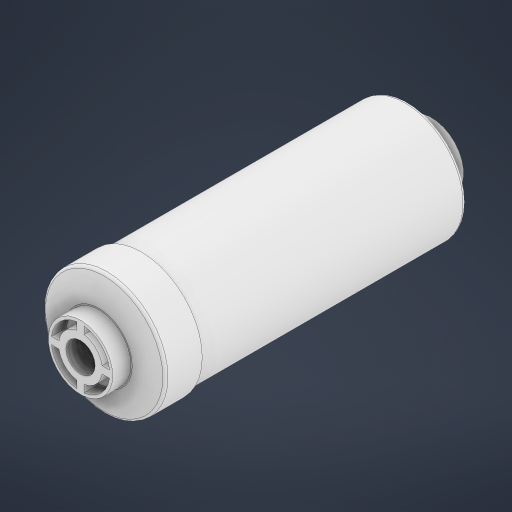
# Autodesk Inventor part: 2x6 Air Tank
Saved by Autodesk Inventor 2024 (Build 280153000, 153)
## iProperties
Created: 2024-02-04
Part Number: 2x6 Air Tank
Material: Generic
Document SubType Name: Modeling
Designer: Juan
Density: 1 g/cm^3
Appearance: Smooth - White
Author: Juan
Autodesk Inventor part; units mm, degrees
ref_plane "YZ Plane" through (0, 0, 0) normal (1, 0, 0) x (0, 1, 0)
ref_plane "XZ Plane" through (0, 0, 0) normal (0, 1, 0) x (-1, 0, 0)
ref_plane "XY Plane" through (0, 0, 0) normal (0, 0, 1) x (1, 0, 0)
sketch "Sketch1" plane through (0, 0, 0) normal (0, 0, 1) x (1, 0, 0)
  circle A0 centre (0, 0) radius 26.4795
  dimension "d0" = 52.959
  constraints: 1 centre point, 1 coincident
  measures "d0" diameter of A0
extrude "Extrusion1" add sketch "Sketch1" along normal blind 152.4
sketch "Sketch2" plane through (0, 0, 152.4) normal (0, 0, 1) x (1, 0, 0)
  circle A0 centre (0, 0) radius 13.97
  circle A1 centre (0, 0) radius 26.4795
  dimension "d3" = 27.94
  constraints: 2 centre point, 2 coincident
  measures "d3" diameter of A0
extrude "Extrusion2" cut sketch "Sketch2" against normal blind 7.9248
sketch "Sketch3" plane through (0, 0, 0) normal (0, 0, -1) x (-1, 0, 0)
  circle A0 centre (0, 0) radius 13.97
  circle A1 centre (0, 0) radius 26.4795
  dimension "d6" = 27.94
  constraints: 2 centre point, 2 coincident
  measures "d6" diameter of A0
extrude "Extrusion3" cut sketch "Sketch3" against normal blind 7.9248
sketch "Sketch4" plane through (0, 0, 7.9248) normal (0, 0, -1) x (-1, 0, 0)
  circle A0 centre (0, 0) radius 13.97 projected
  circle A1 centre (0, 0) radius 25.2095
  circle A2 centre (0, 0) radius 26.4795
  dimension "d9" = 50.419
  constraints: 2 centre point, 2 coincident
  measures "d9" diameter of A1
extrude "Extrusion4" cut sketch "Sketch4" against normal blind 116.84 contours A2
fillet "Fillet1" radius 1.27 1 edges at (-26.4795, 0, 124.7648)
chamfer "Chamfer1" distance 2.54 angle 78 1 edges at (-26.4795, 0, 144.4752) measured on face at (26.3936, -2.1307, 138.3282)
fillet "Fillet2" radius 1.27 1 edges at (-26.4795, 0, 141.9352)
chamfer "Chamfer2" distance 2.54 angle 77 1 edges at (25.2095, 0, 7.9248) measured on face at (-24.883, -4.0439, 85.8181)
fillet "Fillet3" radius 1.27 1 edges at (25.2095, 0, 10.4648)
sketch "Sketch6" plane through (0, 0, 152.4) normal (0, 0, 1) x (1, 0, 0)
  circle A0 centre (0, 0) radius 6.35
  dimension "d23" = 12.7
  constraints: 1 centre point, 1 coincident
  measures "d23" diameter of A0
extrude "Extrusion6" cut sketch "Sketch6" against normal through all
sketch "Sketch7" plane through (0, 0, 7.9248) normal (0, 0, -1) x (-1, 0, 0)
  circle A0 centre (0, 0) radius 22.225
  dimension "d26" = 44.45
  constraints: 1 centre point, 1 coincident
  measures "d26" diameter of A0
sketch "Sketch8" plane through (0, 0, 0) normal (0, 0, -1) x (-1, 0, 0)
  circle A0 centre (0, 0) radius 1.3033
  constraints: 1 centre point, 1 coincident
extrude "Extrusion7" add sketch "Sketch8" against normal blind 76.2
sketch "Sketch9" plane through (0, 0, 76.2) normal (0, 0, 1) x (1, 0, 0)
  circle A0 centre (0, 0) radius 1.3033 projected
  circle A1 centre (0, 0) radius 22.225
  dimension "d29" = 44.45
  constraints: 1 centre point, 1 coincident
  measures "d29" diameter of A1
extrude "Extrusion8" cut sketch "Sketch9" along normal blind 63.5 and the other way blind 63.5
sketch "Sketch10" plane through (0, 0, 0) normal (0, 0, -1) x (-1, 0, 0)
  circle A0 centre (0, 0) radius 1.9784
  constraints: 1 centre point, 1 coincident
extrude "Extrusion9" cut sketch "Sketch10" against normal through all
thread "Thread1" size "1/2-13 UNC" class "2B" standard "ANSI Unified Screw Threads" length 18.2626
thread "Thread2" size "1/2-13 UNC" class "2B" standard "ANSI Unified Screw Threads" length 18.2626
sketch "Sketch11" plane through (0, 0, 152.4) normal (0, 0, 1) x (1, 0, 0)
  circle A0 centre (0, 0) radius 12.7
  circle A1 centre (0, 0) radius 9.525
  circle A2 centre (0, 9.525) radius 1.5875
  circle A3 centre (9.525, 0) radius 1.5875
  circle A4 centre (0, -9.525) radius 1.5875
  circle A5 centre (-9.525, 0) radius 1.5875
  line L0 (-13.6194, 1.5875) -> (-8.6056, 1.5875)
  line L1 (-8.6056, 1.5875) -> (-8.6056, -1.5875)
  line L2 (-8.6056, -1.5875) -> (-13.6194, -1.5875)
  line L3 (-13.6194, -1.5875) -> (-13.6194, 1.5875)
  line L4 (-13.6194, 1.5875) -> (-8.6056, -1.5875) construction
  line L5 (-8.6056, 1.5875) -> (-13.6194, -1.5875) construction
  line L6 (6.086, 1.5875) -> (12.964, 1.5875)
  line L7 (12.964, 1.5875) -> (12.964, -1.5875)
  line L8 (12.964, -1.5875) -> (6.086, -1.5875)
  line L9 (6.086, -1.5875) -> (6.086, 1.5875)
  line L10 (6.086, 1.5875) -> (12.964, -1.5875) construction
  line L11 (12.964, 1.5875) -> (6.086, -1.5875) construction
  line L12 (-1.5875, -6.1744) -> (1.5875, -6.1744)
  line L13 (1.5875, -6.1744) -> (1.5875, -12.8756)
  line L14 (1.5875, -12.8756) -> (-1.5875, -12.8756)
  line L15 (-1.5875, -12.8756) -> (-1.5875, -6.1744)
  line L16 (-1.5875, -6.1744) -> (1.5875, -12.8756) construction
  line L17 (1.5875, -6.1744) -> (-1.5875, -12.8756) construction
  circle A6 centre (0, 0) radius 6.35 projected
  line L18 (-1.5875, 12.9016) -> (1.5875, 12.9016)
  line L19 (1.5875, 12.9016) -> (1.5875, 6.1484)
  line L20 (1.5875, 6.1484) -> (-1.5875, 6.1484)
  line L21 (-1.5875, 6.1484) -> (-1.5875, 12.9016)
  line L22 (-1.5875, 12.9016) -> (1.5875, 6.1484) construction
  line L23 (1.5875, 12.9016) -> (-1.5875, 6.1484) construction
  point P0 (-11.1125, 0)
  point P1 (-1.5875, -9.3918)
  point P2 (-9.3918, -1.5875)
  point P3 (-12.6004, -1.5875)
  point P4 (-1.5875, -12.6004)
  point P5 (1.5875, -12.6004)
  point P6 (12.6004, -1.5875)
  point P7 (9.3918, -1.5875)
  point P8 (1.5875, -9.3918)
  point P9 (1.5875, 9.3918)
  point P10 (9.3918, 1.5875)
  point P11 (12.6004, 1.5875)
  point P12 (1.5875, 12.6004)
  point P13 (-1.5875, 12.6004)
  point P14 (-12.6004, 1.5875)
  point P15 (-9.3918, 1.5875)
  point P16 (-1.5875, 9.3918)
  dimension "d45" = 3.175
  dimension "d40" = 25.4
  dimension "d41" = 19.05
  dimension "d42" = 3.175
  dimension "d43" = 3.175
  dimension "d44" = 3.175
  constraints: 48 end point, 8 midpoint, 8 parallel, 5 centre point, 4 horizontal, 4 perpendicular, 4 point on circle, 2 coincident, 2 point on line, 1 horizontal alignment, 4 other
  measures "d40" diameter of A0
  measures "d41" diameter of A1
  measures "d42" diameter of A2
  measures "d43" diameter of A3
  measures "d44" diameter of A4
extrude "Extrusion10" cut sketch "Sketch11" against normal blind 6.35 contours L6 A1 L19 A0 | A0 L13 A1 L8 | L21 A1 L0 A0 | A0 L2 A1 L15
sketch "Sketch12" plane through (0, 0, 0) normal (0, 0, -1) x (-1, 0, 0)
  circle A0 centre (0, 0) radius 12.7
  line L0 (12.6004, -1.5875) -> (9.3918, -1.5875) projected
  circle A1 centre (0, 0) radius 9.525
  line L1 (-1.5875, 5.8819) -> (1.5875, 5.8819)
  line L2 (1.5875, 5.8819) -> (1.5875, 13.1681)
  line L3 (1.5875, 13.1681) -> (-1.5875, 13.1681)
  line L4 (-1.5875, 13.1681) -> (-1.5875, 5.8819)
  line L5 (-1.5875, 5.8819) -> (1.5875, 13.1681) construction
  line L6 (1.5875, 5.8819) -> (-1.5875, 13.1681) construction
  line L7 (5.4881, 1.5875) -> (13.5619, 1.5875)
  line L8 (13.5619, 1.5875) -> (13.5619, -1.5875)
  line L9 (13.5619, -1.5875) -> (5.4881, -1.5875)
  line L10 (5.4881, -1.5875) -> (5.4881, 1.5875)
  line L11 (5.4881, 1.5875) -> (13.5619, -1.5875) construction
  line L12 (13.5619, 1.5875) -> (5.4881, -1.5875) construction
  line L13 (-1.5875, -5.9212) -> (1.5875, -5.9212)
  line L14 (1.5875, -5.9212) -> (1.5875, -13.1288)
  line L15 (1.5875, -13.1288) -> (-1.5875, -13.1288)
  line L16 (-1.5875, -13.1288) -> (-1.5875, -5.9212)
  line L17 (-1.5875, -5.9212) -> (1.5875, -13.1288) construction
  line L18 (1.5875, -5.9212) -> (-1.5875, -13.1288) construction
  line L19 (-12.9783, 1.5875) -> (-6.0717, 1.5875)
  line L20 (-6.0717, 1.5875) -> (-6.0717, -1.5875)
  line L21 (-6.0717, -1.5875) -> (-12.9783, -1.5875)
  line L22 (-12.9783, -1.5875) -> (-12.9783, 1.5875)
  line L23 (-12.9783, 1.5875) -> (-6.0717, -1.5875) construction
  line L24 (-6.0717, 1.5875) -> (-12.9783, -1.5875) construction
  point P0 (0, 9.525)
  point P1 (9.525, 0)
  point P2 (0, -9.525)
  point P3 (-9.525, 0)
  point P4 (1.5875, -9.3918)
  point P5 (1.5875, -12.6004)
  point P6 (-9.3918, -1.5875)
  point P7 (-12.6004, -1.5875)
  point P8 (-1.5875, -12.6004)
  point P9 (-1.5875, -9.3918)
  point P10 (9.3918, 1.5875)
  point P11 (12.6004, 1.5875)
  point P12 (1.5875, 12.6004)
  point P13 (1.5875, 9.3918)
  point P14 (-12.6004, 1.5875)
  point P15 (-9.3918, 1.5875)
  point P16 (-1.5875, 9.3918)
  point P17 (-1.5875, 12.6004)
  constraints: 48 end point, 8 midpoint, 8 parallel, 5 point on circle, 4 horizontal, 4 perpendicular, 2 coincident, 2 point on line, 1 centre point, 2 other
extrude "Extrusion11" cut sketch "Sketch12" against normal blind 6.35 contours A0 L14 A1 L0 | L7 A1 L2 A0 | A0 L21 A1 L16 | L4 A1 L19 A0
body "Solid1"
